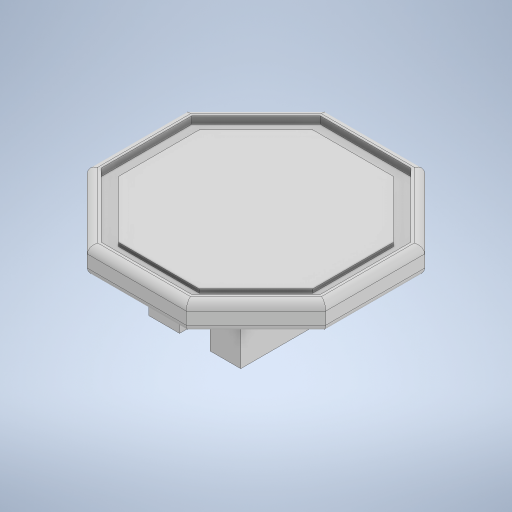
# Autodesk Inventor part: OV-PAM_bottom_2
Saved by Autodesk Inventor 2024 (Build 280153000, 153)
## iProperties
Created: 2023-06-16
Part Number: OV-PAM_bottom_2
Material: 일반
Document SubType Name: Modeling
Designer: jsw
Density: 1 g/cm^3
Appearance: 기본값
Author: jsw
Autodesk Inventor part; units mm, degrees
ref_plane "YZ Plane" through (0, 0, 0) normal (1, 0, 0) x (0, 1, 0)
ref_plane "XZ Plane" through (0, 0, 0) normal (0, 1, 0) x (-1, 0, 0)
ref_plane "XY Plane" through (0, 0, 0) normal (0, 0, 1) x (1, 0, 0)
sketch "스케치3" plane through (0, 0, 0) normal (0, 1, 0) x (-1, 0, 0)
  line L0 (19.4959, -8.0755) -> (8.0755, -19.4959)
  line L1 (8.0755, -19.4959) -> (-8.0755, -19.4959)
  line L2 (-8.0755, -19.4959) -> (-19.4959, -8.0755)
  line L3 (-19.4959, -8.0755) -> (-19.4959, 8.0755)
  line L4 (-19.4959, 8.0755) -> (-8.0755, 19.4959)
  line L5 (-8.0755, 19.4959) -> (8.0755, 19.4959)
  line L6 (8.0755, 19.4959) -> (19.4959, 8.0755)
  line L7 (19.4959, 8.0755) -> (19.4959, -8.0755)
  line L8 (6.75, -16.2959) -> (-6.75, -16.2959)
  line L9 (-6.75, -16.2959) -> (-16.2959, -6.75)
  line L10 (-16.2959, -6.75) -> (-16.2959, 6.75)
  line L11 (-16.2959, 6.75) -> (-6.75, 16.2959)
  line L12 (-6.75, 16.2959) -> (6.75, 16.2959)
  line L13 (6.75, 16.2959) -> (16.2959, 6.75)
  line L14 (16.2959, 6.75) -> (16.2959, -6.75)
  line L15 (16.2959, -6.75) -> (6.75, -16.2959)
  point P0 (0, 0)
  point P1 (0, 0)
  point P2 (0, 0)
  point P3 (0, 0)
  dimension "d66" = 13.5
  dimension "d67" = 3.2
  constraints: 32 end point, 3 coincident, 2 horizontal, 34 other
  measures "d66" distance of L8.start L8.end
  measures "d67" distance between parallel lines of L15 L0
extrude "돌출2" add sketch "스케치3" along normal blind 4.4 contours L0 L1 L2 L3 L4 L5 L6 L7 | L8 L9 L10 L11 L12 L13 L14 L15
sketch "스케치9" plane through (0, 0, 0) normal (0, -1, 0) x (1, 0, 0)
  line L0 (7.5, 10) -> (2.5, 10)
  line L1 (2.5, 10) -> (2.5, -10)
  line L2 (2.5, -10) -> (7.5, -10)
  line L3 (7.5, -10) -> (7.5, 10)
  line L4 (7.5, 10) -> (2.5, -10) construction
  line L5 (2.5, 10) -> (7.5, -10) construction
  line L6 (-2.5, 10) -> (-7.5, 10)
  line L7 (-7.5, 10) -> (-7.5, -10)
  line L8 (-7.5, -10) -> (-2.5, -10)
  line L9 (-2.5, 10) -> (-7.5, -10) construction
  line L10 (-7.5, 10) -> (-2.5, -10) construction
  line L11 (-2.5, -10) -> (-2.5, 10)
  point P0 (0, 0)
  point P1 (5, 0)
  point P2 (-5, 0)
  dimension "d42" = 20
  dimension "d43" = 5
  dimension "d44" = 2.5
  dimension "d47" = 10
  constraints: 24 end point, 2 horizontal, 2 midpoint, 2 parallel, 1 collinear, 1 horizontal alignment, 1 perpendicular, 10 other
  measures "d42" distance of L2.end L0.start
  measures "d43" distance of L1.end L2.end
  measures "d44" distance from line of L1 point (0, 0)
  measures "d47" distance of L0.start L6.start
extrude "돌출8" add sketch "스케치9" along normal blind 10
sketch "스케치10" plane through (-7.5, 0, -10) normal (-1, 0, 0) x (0, 0, 1)
  circle A0 centre (15, -5) radius 1.25
  line L0 (19.9591, 0) -> (0.0886, 0)
  line L1 (18.0755, 0) -> (1.9245, 0) projected
  circle A1 centre (5, -5) radius 1.25
  line L2 (20, 0) -> (20, -10) projected
  point P0 (10, 0)
  dimension "d54" = 2.5
  dimension "d57" = 10
  dimension "d62" = 5
  dimension "d63" = 5
  constraints: 2 centre point, 2 end point, 1 horizontal, 1 point on line, 2 other
  measures "d54" diameter of A0
  measures "d57" distance of A0.centre A1.centre
  measures "d62" distance from line of L0 A0.centre
  measures "d63" distance from line of L2 A0.centre
extrude "돌출9" cut sketch "스케치10" against normal blind 20
fillet "모깎기1" radius 1.2 16 edges at (-13.7857, 4.4, 13.7857) (0, 4.4, 19.4959) (13.7857, 4.4, 13.7857) (19.4959, 4.4, 0) (13.7857, 4.4, -13.7857) (0, 4.4, -19.4959) (-13.7857, 4.4, -13.7857) (-19.4959, 4.4, 0) (-13.7857, 0, 13.7857) (0, 0, 19.4959) (13.7857, 0, 13.7857) (19.4959, 0, 0) (13.7857, 0, -13.7857) (0, 0, -19.4959) (-13.7857, 0, -13.7857) (-19.4959, 0, 0)
sketch "스케치12" plane through (0, 4.4, 0) normal (0, 1, 0) x (1, 0, 0)
  line L0 (7.4127, -17.8959) -> (-7.4127, -17.8959)
  line L1 (-7.4127, -17.8959) -> (-17.8959, -7.4127)
  line L2 (-17.8959, -7.4127) -> (-17.8959, 7.4127)
  line L3 (-17.8959, 7.4127) -> (-7.4127, 17.8959)
  line L4 (-7.4127, 17.8959) -> (7.4127, 17.8959)
  line L5 (7.4127, 17.8959) -> (17.8959, 7.4127)
  line L6 (17.8959, 7.4127) -> (17.8959, -7.4127)
  line L7 (17.8959, -7.4127) -> (7.4127, -17.8959)
  line L8 (-6.5843, 15.8959) -> (6.5843, 15.8959)
  line L9 (6.5843, 15.8959) -> (15.8959, 6.5843)
  line L10 (15.8959, 6.5843) -> (15.8959, -6.5843)
  line L11 (15.8959, -6.5843) -> (6.5843, -15.8959)
  line L12 (6.5843, -15.8959) -> (-6.5843, -15.8959)
  line L13 (-6.5843, -15.8959) -> (-15.8959, -6.5843)
  line L14 (-15.8959, -6.5843) -> (-15.8959, 6.5843)
  line L15 (-15.8959, 6.5843) -> (-6.5843, 15.8959)
  line L16 (-18.2959, -7.5784) -> (-18.2959, 7.5784) projected
  line L17 (-19.4959, 8.0755) -> (-19.4959, -8.0755) projected
  point P0 (0, 0)
  point P1 (0, 0)
  point P2 (0, 0)
  point P3 (-17.8959, 0)
  point P4 (-19.4959, 0)
  point P5 (-15.8959, 0)
  dimension "d100" = 1.6
  dimension "d101" = 2
  constraints: 32 end point, 3 midpoint, 2 coincident, 2 horizontal, 34 other
  measures "d100" distance of point (-17.896, 0) point (-19.496, 0)
  measures "d101" distance from line of point (-15.896, 0) L2
extrude "돌출11" cut sketch "스케치12" against normal blind 1.2
sketch "스케치13" plane through (0, 4.4, 0) normal (0, 1, 0) x (1, 0, 0)
  line L0 (15.8959, 6.5843) -> (6.5843, 15.8959) projected
  line L1 (6.5843, 15.8959) -> (-6.5843, 15.8959) projected
  line L2 (-6.5843, 15.8959) -> (-15.8959, 6.5843) projected
  line L3 (-15.8959, 6.5843) -> (-15.8959, -6.5843) projected
  line L4 (-15.8959, -6.5843) -> (-6.5843, -15.8959) projected
  line L5 (-6.5843, -15.8959) -> (6.5843, -15.8959) projected
  line L6 (6.5843, -15.8959) -> (15.8959, -6.5843) projected
  line L7 (15.8959, -6.5843) -> (15.8959, 6.5843) projected
  point P0 (0, 0)
extrude "돌출12" cut sketch "스케치13" against normal blind 0.6
